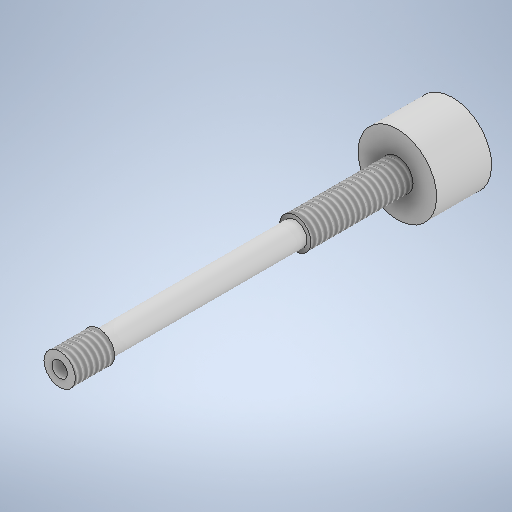
# Autodesk Inventor part: HeatBreak_HotEnd
Saved by Autodesk Inventor 2025.2 (Build 292293000, 293)
## iProperties
Created: 2026-06-11
Part Number: HeatBreak_HotEnd
Material: Generic
Document SubType Name: Modeling
Designer: Simon
Density: 1 g/cm^3
Appearance: Default
Author: Simon
Autodesk Inventor part; units mm, degrees
ref_plane "YZ Plane" through (0, 0, 0) normal (1, 0, 0) x (0, 1, 0)
ref_plane "XZ Plane" through (0, 0, 0) normal (0, 1, 0) x (-1, 0, 0)
ref_plane "XY Plane" through (0, 0, 0) normal (0, 0, 1) x (1, 0, 0)
sketch "Sketch1" plane through (0, 0, 0) normal (1, 0, 0) x (0, 1, 0)
  line L0 (0, 0) -> (1, 0)
  line L1 (1, 0) -> (1, -50)
  line L2 (1, -50) -> (0, -50)
  line L3 (0, -50) -> (0, 0)
  line L4 (0, -50) -> (3, -50)
  line L5 (3, -50) -> (3, -45)
  line L6 (0, -50) -> (5, -50)
  line L7 (5, -50) -> (5, -45)
  line L8 (5, -45) -> (0, -45)
  line L9 (5, -45) -> (5, -43)
  line L10 (5, -43) -> (0, -43)
  line L11 (0, -43) -> (2, -43)
  line L12 (2, -43) -> (2, -30)
  line L13 (2, -30) -> (0, -30)
  line L14 (0, -30) -> (1.5, -30)
  line L15 (1.5, -30) -> (1.5, -5)
  line L16 (1.5, -5) -> (0, -5)
  line L17 (0, -5) -> (2, -5)
  line L18 (2, -5) -> (2, 0)
  line L19 (2, 0) -> (0, 0)
  point P0 (1, -45)
  dimension "d0" = 1
  dimension "d1" = 50
  dimension "d2" = 3
  dimension "d3" = 5
  dimension "d4" = 5
  dimension "d5" = 2
  dimension "d6" = 2
  dimension "d7" = 13
  dimension "d8" = 1.5
  dimension "d9" = 25
  dimension "d10" = 5
  constraints: 40 end point, 13 perpendicular, 8 point on line, 3 horizontal, 1 vertical
  measures "d0" distance of L0.start L0.end
  measures "d1" distance of L0.end L1.end
  measures "d2" distance of L2.end L4.end
  measures "d3" distance of L4.end L5.end
  measures "d4" distance of L2.end L6.end
  measures "d5" distance of L7.end L9.end
  measures "d6" distance of L10.end L11.end
  measures "d7" distance of L11.end L12.end
  measures "d8" distance of L13.end L14.end
  measures "d9" distance of L14.end L15.end
  measures "d10" distance of L17.end L18.end
revolve "Revolution1" add sketch "Sketch1" angle 360 about axis through (0, 0, -50) along (0, 0, 1) contours L19 L18 L17 L16 L1 | L16 L15 L13 L1 | L13 L12 L10 L1 | L10 L9 L8 L1 | L8 L7 L6 L5
thread "Thread1" size "M4x0.7" class "6g" standard "ISO Metric profile" full length
thread "Thread2" size "M4x0.7" class "6g" standard "ANSI Metric M Profile" full length
thread "Thread3" size "M6x1" class "6H" standard "ANSI Metric M Profile" full length
body "Solid1"
